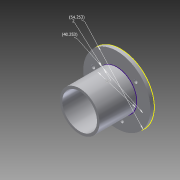
# Autodesk Inventor part: SzenzorSzuportKerek
Saved by Autodesk Inventor 2015 SP1 (Build 190203100, 203)
## iProperties
Created: 2014-11-14
Part Number: SzenzorSzuportKerek
Material: PPS Plastic
Document SubType Name: Modeling
Designer: laca
Density: 1.637 g/cm^3
Appearance: Smooth - White
Mass: 17.5167 g
Surface Area: 98.5038 cm^2
Volume: 10.7005 cm^3
Author: laca
Autodesk Inventor part; units mm, degrees
ref_plane "YZ Plane" through (0, 0, 0) normal (1, 0, 0) x (0, 1, 0)
ref_plane "XZ Plane" through (0, 0, 0) normal (0, 1, 0) x (-1, 0, 0)
ref_plane "XY Plane" through (0, 0, 0) normal (0, 0, 1) x (1, 0, 0)
sketch "Sketch9" plane through (0, 0, -8.5889) normal (0, 0, 1) x (0.9992, 0.041, 0)
  circle A0 centre (0, 0) radius 27.1267
  circle A1 centre (0, 0) radius 20.1267
  circle A2 centre (-18.793, 7.2047) radius 1.5
  circle A3 centre (3.157, -19.8775) radius 1.5
  circle A4 centre (-7.3961, 16.9572) radius 3
  circle A5 centre (-7.3961, 16.9572) radius 3
  circle A6 centre (15.6359, 12.6728) radius 1.5
  dimension "d13" = 40.2533
  dimension "d14" = 54.2533
  measures "d14" diameter of A0
extrude "Extrusion1" add sketch "Sketch9" along normal blind 3 contours A0 | A1 A3 A2 A4 A6 | A6 A1 | A1 A6 | A3 A1 | A1 A3 | A4 A1 | A1 A4 | A2 A1 | A1 A2
sketch "Sketch2" plane through (0, 0, -5.5889) normal (0, 0, 1) x (1, 0, 0)
  circle A0 centre (0, 0) radius 16
  circle A1 centre (0, 0) radius 14
  dimension "d3" = 32
  dimension "d6" = 2
  constraints: 2 centre point, 2 coincident
  measures "d3" diameter of A0
  measures "d6" radial gap between concentric circles of A0 A1
extrude "Extrusion3" add sketch "Sketch2" along normal blind 30
extrude "Extrusion4" cut sketch "Sketch2" against normal through all contours A1
extrude "Extrusion5" cut sketch "Sketch9" along normal through all contours A6 A1 | A1 A6 | A3 A1 | A1 A3 | A2 A1 | A1 A2
body "Solid1"
